Autodesk Inventor part; units mm, degrees
(part 6 of 13)
  spline S758 degree 3 poles (41.4277, 33.5866) (41.4277, 33.0506) (41.8622, 32.616) (42.3982, 32.616) knots 0 0 0 0 1 1 1 1
  line L2394 (41.4277, 33.5866) -> (41.4277, 33.0506) construction
  line L2395 (41.4277, 33.0506) -> (41.8622, 32.616) construction
  line L2396 (41.8622, 32.616) -> (42.3982, 32.616) construction
  spline S759 degree 3 poles (42.3982, 32.616) (42.9342, 32.616) (43.3688, 33.0506) (43.3688, 33.5866) knots 0 0 0 0 1 1 1 1
  line L2397 (42.3982, 32.616) -> (42.9342, 32.616) construction
  line L2398 (42.9342, 32.616) -> (43.3688, 33.0506) construction
  line L2399 (43.3688, 33.0506) -> (43.3688, 33.5866) construction
  spline S760 degree 3 poles (45.9229, 33.5866) (45.9229, 34.1226) (45.4883, 34.5571) (44.9523, 34.5571) knots 0 0 0 0 1 1 1 1
  line L2400 (45.9229, 33.5866) -> (45.9229, 34.1226) construction
  line L2401 (45.9229, 34.1226) -> (45.4883, 34.5571) construction
  line L2402 (45.4883, 34.5571) -> (44.9523, 34.5571) construction
  spline S761 degree 3 poles (44.9523, 34.5571) (44.4163, 34.5571) (43.9818, 34.1226) (43.9818, 33.5866) knots 0 0 0 0 1 1 1 1
  line L2403 (44.9523, 34.5571) -> (44.4163, 34.5571) construction
  line L2404 (44.4163, 34.5571) -> (43.9818, 34.1226) construction
  line L2405 (43.9818, 34.1226) -> (43.9818, 33.5866) construction
  spline S762 degree 3 poles (43.9818, 33.5866) (43.9818, 33.0506) (44.4163, 32.616) (44.9523, 32.616) knots 0 0 0 0 1 1 1 1
  line L2406 (43.9818, 33.5866) -> (43.9818, 33.0506) construction
  line L2407 (43.9818, 33.0506) -> (44.4163, 32.616) construction
  line L2408 (44.4163, 32.616) -> (44.9523, 32.616) construction
  spline S763 degree 3 poles (44.9523, 32.616) (45.4883, 32.616) (45.9229, 33.0506) (45.9229, 33.5866) knots 0 0 0 0 1 1 1 1
  line L2409 (44.9523, 32.616) -> (45.4883, 32.616) construction
  line L2410 (45.4883, 32.616) -> (45.9229, 33.0506) construction
  line L2411 (45.9229, 33.0506) -> (45.9229, 33.5866) construction
  spline S764 degree 3 poles (34.4294, 0.3832) (34.4294, 0.9191) (33.9948, 1.3537) (33.4588, 1.3537) knots 0 0 0 0 1 1 1 1
  line L2412 (34.4294, 0.3832) -> (34.4294, 0.9191) construction
  line L2413 (34.4294, 0.9191) -> (33.9948, 1.3537) construction
  line L2414 (33.9948, 1.3537) -> (33.4588, 1.3537) construction
  spline S765 degree 3 poles (33.4588, 1.3537) (32.9228, 1.3537) (32.4883, 0.9191) (32.4883, 0.3832) knots 0 0 0 0 1 1 1 1
  line L2415 (33.4588, 1.3537) -> (32.9228, 1.3537) construction
  line L2416 (32.9228, 1.3537) -> (32.4883, 0.9191) construction
  line L2417 (32.4883, 0.9191) -> (32.4883, 0.3832) construction
  spline S766 degree 3 poles (32.4883, 0.3832) (32.4883, -0.1529) (32.9228, -0.5874) (33.4588, -0.5874) knots 0 0 0 0 1 1 1 1
  line L2418 (32.4883, 0.3832) -> (32.4883, -0.1529) construction
  line L2419 (32.4883, -0.1529) -> (32.9228, -0.5874) construction
  line L2420 (32.9228, -0.5874) -> (33.4588, -0.5874) construction
  spline S767 degree 3 poles (33.4588, -0.5874) (33.9948, -0.5874) (34.4294, -0.1529) (34.4294, 0.3832) knots 0 0 0 0 1 1 1 1
  line L2421 (33.4588, -0.5874) -> (33.9948, -0.5874) construction
  line L2422 (33.9948, -0.5874) -> (34.4294, -0.1529) construction
  line L2423 (34.4294, -0.1529) -> (34.4294, 0.3832) construction
  spline S768 degree 3 poles (31.8752, 0.3832) (31.8752, 0.9191) (31.4407, 1.3537) (30.9047, 1.3537) knots 0 0 0 0 1 1 1 1
  line L2424 (31.8752, 0.3832) -> (31.8752, 0.9191) construction
  line L2425 (31.8752, 0.9191) -> (31.4407, 1.3537) construction
  line L2426 (31.4407, 1.3537) -> (30.9047, 1.3537) construction
  spline S769 degree 3 poles (30.9047, 1.3537) (30.3687, 1.3537) (29.9342, 0.9191) (29.9342, 0.3832) knots 0 0 0 0 1 1 1 1
  line L2427 (30.9047, 1.3537) -> (30.3687, 1.3537) construction
  line L2428 (30.3687, 1.3537) -> (29.9342, 0.9191) construction
  line L2429 (29.9342, 0.9191) -> (29.9342, 0.3832) construction
  spline S770 degree 3 poles (29.9342, 0.3832) (29.9342, -0.1529) (30.3687, -0.5874) (30.9047, -0.5874) knots 0 0 0 0 1 1 1 1
  line L2430 (29.9342, 0.3832) -> (29.9342, -0.1529) construction
  line L2431 (29.9342, -0.1529) -> (30.3687, -0.5874) construction
  line L2432 (30.3687, -0.5874) -> (30.9047, -0.5874) construction
  spline S771 degree 3 poles (30.9047, -0.5874) (31.4407, -0.5874) (31.8752, -0.1529) (31.8752, 0.3832) knots 0 0 0 0 1 1 1 1
  line L2433 (30.9047, -0.5874) -> (31.4407, -0.5874) construction
  line L2434 (31.4407, -0.5874) -> (31.8752, -0.1529) construction
  line L2435 (31.8752, -0.1529) -> (31.8752, 0.3832) construction
  spline S772 degree 3 poles (29.3211, 0.3832) (29.3211, 0.9191) (28.8866, 1.3537) (28.3506, 1.3537) knots 0 0 0 0 1 1 1 1
  line L2436 (29.3211, 0.3832) -> (29.3211, 0.9191) construction
  line L2437 (29.3211, 0.9191) -> (28.8866, 1.3537) construction
  line L2438 (28.8866, 1.3537) -> (28.3506, 1.3537) construction
  spline S773 degree 3 poles (28.3506, 1.3537) (27.8146, 1.3537) (27.3801, 0.9191) (27.3801, 0.3832) knots 0 0 0 0 1 1 1 1
  line L2439 (28.3506, 1.3537) -> (27.8146, 1.3537) construction
  line L2440 (27.8146, 1.3537) -> (27.3801, 0.9191) construction
  line L2441 (27.3801, 0.9191) -> (27.3801, 0.3832) construction
  spline S774 degree 3 poles (27.3801, 0.3832) (27.3801, -0.1529) (27.8146, -0.5874) (28.3506, -0.5874) knots 0 0 0 0 1 1 1 1
  line L2442 (27.3801, 0.3832) -> (27.3801, -0.1529) construction
  line L2443 (27.3801, -0.1529) -> (27.8146, -0.5874) construction
  line L2444 (27.8146, -0.5874) -> (28.3506, -0.5874) construction
  spline S775 degree 3 poles (28.3506, -0.5874) (28.8866, -0.5874) (29.3211, -0.1529) (29.3211, 0.3832) knots 0 0 0 0 1 1 1 1
  line L2445 (28.3506, -0.5874) -> (28.8866, -0.5874) construction
  line L2446 (28.8866, -0.5874) -> (29.3211, -0.1529) construction
  line L2447 (29.3211, -0.1529) -> (29.3211, 0.3832) construction
  spline S776 degree 3 poles (43.3688, 0.3832) (43.3688, 0.9191) (42.9342, 1.3537) (42.3982, 1.3537) knots 0 0 0 0 1 1 1 1
  line L2448 (43.3688, 0.3832) -> (43.3688, 0.9191) construction
  line L2449 (43.3688, 0.9191) -> (42.9342, 1.3537) construction
  line L2450 (42.9342, 1.3537) -> (42.3982, 1.3537) construction
  spline S777 degree 3 poles (42.3982, 1.3537) (41.8622, 1.3537) (41.4277, 0.9191) (41.4277, 0.3832) knots 0 0 0 0 1 1 1 1
  line L2451 (42.3982, 1.3537) -> (41.8622, 1.3537) construction
  line L2452 (41.8622, 1.3537) -> (41.4277, 0.9191) construction
  line L2453 (41.4277, 0.9191) -> (41.4277, 0.3832) construction
  spline S778 degree 3 poles (41.4277, 0.3832) (41.4277, -0.1529) (41.8622, -0.5874) (42.3982, -0.5874) knots 0 0 0 0 1 1 1 1
  line L2454 (41.4277, 0.3832) -> (41.4277, -0.1529) construction
  line L2455 (41.4277, -0.1529) -> (41.8622, -0.5874) construction
  line L2456 (41.8622, -0.5874) -> (42.3982, -0.5874) construction
  spline S779 degree 3 poles (42.3982, -0.5874) (42.9342, -0.5874) (43.3688, -0.1529) (43.3688, 0.3832) knots 0 0 0 0 1 1 1 1
  line L2457 (42.3982, -0.5874) -> (42.9342, -0.5874) construction
  line L2458 (42.9342, -0.5874) -> (43.3688, -0.1529) construction
  line L2459 (43.3688, -0.1529) -> (43.3688, 0.3832) construction
  spline S780 degree 3 poles (35.7064, 2.9373) (35.7064, 3.4732) (35.2719, 3.9078) (34.7358, 3.9078) knots 0 0 0 0 1 1 1 1
  line L2460 (35.7064, 2.9373) -> (35.7064, 3.4732) construction
  line L2461 (35.7064, 3.4732) -> (35.2719, 3.9078) construction
  line L2462 (35.2719, 3.9078) -> (34.7358, 3.9078) construction
  spline S781 degree 3 poles (34.7358, 3.9078) (34.1999, 3.9078) (33.7653, 3.4732) (33.7653, 2.9373) knots 0 0 0 0 1 1 1 1
  line L2463 (34.7358, 3.9078) -> (34.1999, 3.9078) construction
  line L2464 (34.1999, 3.9078) -> (33.7653, 3.4732) construction
  line L2465 (33.7653, 3.4732) -> (33.7653, 2.9373) construction
  spline S782 degree 3 poles (33.7653, 2.9373) (33.7653, 2.4013) (34.1999, 1.9667) (34.7358, 1.9667) knots 0 0 0 0 1 1 1 1
  line L2466 (33.7653, 2.9373) -> (33.7653, 2.4013) construction
  line L2467 (33.7653, 2.4013) -> (34.1999, 1.9667) construction
  line L2468 (34.1999, 1.9667) -> (34.7358, 1.9667) construction
  spline S783 degree 3 poles (34.7358, 1.9667) (35.2719, 1.9667) (35.7064, 2.4013) (35.7064, 2.9373) knots 0 0 0 0 1 1 1 1
  line L2469 (34.7358, 1.9667) -> (35.2719, 1.9667) construction
  line L2470 (35.2719, 1.9667) -> (35.7064, 2.4013) construction
  line L2471 (35.7064, 2.4013) -> (35.7064, 2.9373) construction
  spline S784 degree 3 poles (35.7064, 5.4914) (35.7064, 6.0273) (35.2719, 6.4619) (34.7358, 6.4619) knots 0 0 0 0 1 1 1 1
  line L2472 (35.7064, 5.4914) -> (35.7064, 6.0273) construction
  line L2473 (35.7064, 6.0273) -> (35.2719, 6.4619) construction
  line L2474 (35.2719, 6.4619) -> (34.7358, 6.4619) construction
  spline S785 degree 3 poles (34.7358, 6.4619) (34.1999, 6.4619) (33.7653, 6.0273) (33.7653, 5.4914) knots 0 0 0 0 1 1 1 1
  line L2475 (34.7358, 6.4619) -> (34.1999, 6.4619) construction
  line L2476 (34.1999, 6.4619) -> (33.7653, 6.0273) construction
  line L2477 (33.7653, 6.0273) -> (33.7653, 5.4914) construction
  spline S786 degree 3 poles (33.7653, 5.4914) (33.7653, 4.9554) (34.1999, 4.5208) (34.7358, 4.5208) knots 0 0 0 0 1 1 1 1
  line L2478 (33.7653, 5.4914) -> (33.7653, 4.9554) construction
  line L2479 (33.7653, 4.9554) -> (34.1999, 4.5208) construction
  line L2480 (34.1999, 4.5208) -> (34.7358, 4.5208) construction
  spline S787 degree 3 poles (34.7358, 4.5208) (35.2719, 4.5208) (35.7064, 4.9554) (35.7064, 5.4914) knots 0 0 0 0 1 1 1 1
  line L2481 (34.7358, 4.5208) -> (35.2719, 4.5208) construction
  line L2482 (35.2719, 4.5208) -> (35.7064, 4.9554) construction
  line L2483 (35.7064, 4.9554) -> (35.7064, 5.4914) construction
  spline S788 degree 3 poles (38.2606, 5.4914) (38.2606, 6.0273) (37.826, 6.4619) (37.29, 6.4619) knots 0 0 0 0 1 1 1 1
  line L2484 (38.2606, 5.4914) -> (38.2606, 6.0273) construction
  line L2485 (38.2606, 6.0273) -> (37.826, 6.4619) construction
  line L2486 (37.826, 6.4619) -> (37.29, 6.4619) construction
  spline S789 degree 3 poles (37.29, 6.4619) (36.754, 6.4619) (36.3194, 6.0273) (36.3194, 5.4914) knots 0 0 0 0 1 1 1 1
  line L2487 (37.29, 6.4619) -> (36.754, 6.4619) construction
  line L2488 (36.754, 6.4619) -> (36.3194, 6.0273) construction
  line L2489 (36.3194, 6.0273) -> (36.3194, 5.4914) construction
  spline S790 degree 3 poles (36.3194, 5.4914) (36.3194, 4.9554) (36.754, 4.5208) (37.29, 4.5208) knots 0 0 0 0 1 1 1 1
  line L2490 (36.3194, 5.4914) -> (36.3194, 4.9554) construction
  line L2491 (36.3194, 4.9554) -> (36.754, 4.5208) construction
  line L2492 (36.754, 4.5208) -> (37.29, 4.5208) construction
  spline S791 degree 3 poles (37.29, 4.5208) (37.826, 4.5208) (38.2606, 4.9554) (38.2606, 5.4914) knots 0 0 0 0 1 1 1 1
  line L2493 (37.29, 4.5208) -> (37.826, 4.5208) construction
  line L2494 (37.826, 4.5208) -> (38.2606, 4.9554) construction
  line L2495 (38.2606, 4.9554) -> (38.2606, 5.4914) construction
  spline S792 degree 3 poles (38.2606, 0.3832) (38.2606, 0.9191) (37.826, 1.3537) (37.29, 1.3537) knots 0 0 0 0 1 1 1 1
  line L2496 (38.2606, 0.3832) -> (38.2606, 0.9191) construction
  line L2497 (38.2606, 0.9191) -> (37.826, 1.3537) construction
  line L2498 (37.826, 1.3537) -> (37.29, 1.3537) construction
  spline S793 degree 3 poles (37.29, 1.3537) (36.754, 1.3537) (36.3194, 0.9191) (36.3194, 0.3832) knots 0 0 0 0 1 1 1 1
  line L2499 (37.29, 1.3537) -> (36.754, 1.3537) construction
  line L2500 (36.754, 1.3537) -> (36.3194, 0.9191) construction
  line L2501 (36.3194, 0.9191) -> (36.3194, 0.3832) construction
  spline S794 degree 3 poles (36.3194, 0.3832) (36.3194, -0.1529) (36.754, -0.5874) (37.29, -0.5874) knots 0 0 0 0 1 1 1 1
  line L2502 (36.3194, 0.3832) -> (36.3194, -0.1529) construction
  line L2503 (36.3194, -0.1529) -> (36.754, -0.5874) construction
  line L2504 (36.754, -0.5874) -> (37.29, -0.5874) construction
  spline S795 degree 3 poles (37.29, -0.5874) (37.826, -0.5874) (38.2606, -0.1529) (38.2606, 0.3832) knots 0 0 0 0 1 1 1 1
  line L2505 (37.29, -0.5874) -> (37.826, -0.5874) construction
  line L2506 (37.826, -0.5874) -> (38.2606, -0.1529) construction
  line L2507 (38.2606, -0.1529) -> (38.2606, 0.3832) construction
  spline S796 degree 3 poles (40.8147, 0.3832) (40.8147, 0.9191) (40.3801, 1.3537) (39.8441, 1.3537) knots 0 0 0 0 1 1 1 1
  line L2508 (40.8147, 0.3832) -> (40.8147, 0.9191) construction
  line L2509 (40.8147, 0.9191) -> (40.3801, 1.3537) construction
  line L2510 (40.3801, 1.3537) -> (39.8441, 1.3537) construction
  spline S797 degree 3 poles (39.8441, 1.3537) (39.3081, 1.3537) (38.8735, 0.9191) (38.8735, 0.3832) knots 0 0 0 0 1 1 1 1
  line L2511 (39.8441, 1.3537) -> (39.3081, 1.3537) construction
  line L2512 (39.3081, 1.3537) -> (38.8735, 0.9191) construction
  line L2513 (38.8735, 0.9191) -> (38.8735, 0.3832) construction
  spline S798 degree 3 poles (38.8735, 0.3832) (38.8735, -0.1529) (39.3081, -0.5874) (39.8441, -0.5874) knots 0 0 0 0 1 1 1 1
  line L2514 (38.8735, 0.3832) -> (38.8735, -0.1529) construction
  line L2515 (38.8735, -0.1529) -> (39.3081, -0.5874) construction
  line L2516 (39.3081, -0.5874) -> (39.8441, -0.5874) construction
  spline S799 degree 3 poles (39.8441, -0.5874) (40.3801, -0.5874) (40.8147, -0.1529) (40.8147, 0.3832) knots 0 0 0 0 1 1 1 1
  line L2517 (39.8441, -0.5874) -> (40.3801, -0.5874) construction
  line L2518 (40.3801, -0.5874) -> (40.8147, -0.1529) construction
  line L2519 (40.8147, -0.1529) -> (40.8147, 0.3832) construction
  spline S800 degree 3 poles (38.2606, 2.9373) (38.2606, 3.4732) (37.826, 3.9078) (37.29, 3.9078) knots 0 0 0 0 1 1 1 1
  line L2520 (38.2606, 2.9373) -> (38.2606, 3.4732) construction
  line L2521 (38.2606, 3.4732) -> (37.826, 3.9078) construction
  line L2522 (37.826, 3.9078) -> (37.29, 3.9078) construction
  spline S801 degree 3 poles (37.29, 3.9078) (36.754, 3.9078) (36.3194, 3.4732) (36.3194, 2.9373) knots 0 0 0 0 1 1 1 1
  line L2523 (37.29, 3.9078) -> (36.754, 3.9078) construction
  line L2524 (36.754, 3.9078) -> (36.3194, 3.4732) construction
  line L2525 (36.3194, 3.4732) -> (36.3194, 2.9373) construction
  spline S802 degree 3 poles (36.3194, 2.9373) (36.3194, 2.4013) (36.754, 1.9667) (37.29, 1.9667) knots 0 0 0 0 1 1 1 1
  line L2526 (36.3194, 2.9373) -> (36.3194, 2.4013) construction
  line L2527 (36.3194, 2.4013) -> (36.754, 1.9667) construction
  line L2528 (36.754, 1.9667) -> (37.29, 1.9667) construction
  spline S803 degree 3 poles (37.29, 1.9667) (37.826, 1.9667) (38.2606, 2.4013) (38.2606, 2.9373) knots 0 0 0 0 1 1 1 1
  line L2529 (37.29, 1.9667) -> (37.826, 1.9667) construction
  line L2530 (37.826, 1.9667) -> (38.2606, 2.4013) construction
  line L2531 (38.2606, 2.4013) -> (38.2606, 2.9373) construction
  spline S804 degree 3 poles (35.7064, 8.0455) (35.7064, 8.5815) (35.2719, 9.016) (34.7358, 9.016) knots 0 0 0 0 1 1 1 1
  line L2532 (35.7064, 8.0455) -> (35.7064, 8.5815) construction
  line L2533 (35.7064, 8.5815) -> (35.2719, 9.016) construction
  line L2534 (35.2719, 9.016) -> (34.7358, 9.016) construction
  spline S805 degree 3 poles (34.7358, 9.016) (34.1999, 9.016) (33.7653, 8.5815) (33.7653, 8.0455) knots 0 0 0 0 1 1 1 1
  line L2535 (34.7358, 9.016) -> (34.1999, 9.016) construction
  line L2536 (34.1999, 9.016) -> (33.7653, 8.5815) construction
  line L2537 (33.7653, 8.5815) -> (33.7653, 8.0455) construction
  spline S806 degree 3 poles (33.7653, 8.0455) (33.7653, 7.5095) (34.1999, 7.0749) (34.7358, 7.0749) knots 0 0 0 0 1 1 1 1
  line L2538 (33.7653, 8.0455) -> (33.7653, 7.5095) construction
  line L2539 (33.7653, 7.5095) -> (34.1999, 7.0749) construction
  line L2540 (34.1999, 7.0749) -> (34.7358, 7.0749) construction
  spline S807 degree 3 poles (34.7358, 7.0749) (35.2719, 7.0749) (35.7064, 7.5095) (35.7064, 8.0455) knots 0 0 0 0 1 1 1 1
  line L2541 (34.7358, 7.0749) -> (35.2719, 7.0749) construction
  line L2542 (35.2719, 7.0749) -> (35.7064, 7.5095) construction
  line L2543 (35.7064, 7.5095) -> (35.7064, 8.0455) construction
  spline S808 degree 3 poles (38.2606, 8.0455) (38.2606, 8.5815) (37.826, 9.016) (37.29, 9.016) knots 0 0 0 0 1 1 1 1
  line L2544 (38.2606, 8.0455) -> (38.2606, 8.5815) construction
  line L2545 (38.2606, 8.5815) -> (37.826, 9.016) construction
  line L2546 (37.826, 9.016) -> (37.29, 9.016) construction
  spline S809 degree 3 poles (37.29, 9.016) (36.754, 9.016) (36.3194, 8.5815) (36.3194, 8.0455) knots 0 0 0 0 1 1 1 1
  line L2547 (37.29, 9.016) -> (36.754, 9.016) construction
  line L2548 (36.754, 9.016) -> (36.3194, 8.5815) construction
  line L2549 (36.3194, 8.5815) -> (36.3194, 8.0455) construction
  spline S810 degree 3 poles (36.3194, 8.0455) (36.3194, 7.5095) (36.754, 7.0749) (37.29, 7.0749) knots 0 0 0 0 1 1 1 1
  line L2550 (36.3194, 8.0455) -> (36.3194, 7.5095) construction
  line L2551 (36.3194, 7.5095) -> (36.754, 7.0749) construction
  line L2552 (36.754, 7.0749) -> (37.29, 7.0749) construction
  spline S811 degree 3 poles (37.29, 7.0749) (37.826, 7.0749) (38.2606, 7.5095) (38.2606, 8.0455) knots 0 0 0 0 1 1 1 1
  line L2553 (37.29, 7.0749) -> (37.826, 7.0749) construction
  line L2554 (37.826, 7.0749) -> (38.2606, 7.5095) construction
  line L2555 (38.2606, 7.5095) -> (38.2606, 8.0455) construction
  spline S812 degree 3 poles (35.7064, 10.5996) (35.7064, 11.1356) (35.2719, 11.5701) (34.7358, 11.5701) knots 0 0 0 0 1 1 1 1
  line L2556 (35.7064, 10.5996) -> (35.7064, 11.1356) construction
  line L2557 (35.7064, 11.1356) -> (35.2719, 11.5701) construction
  line L2558 (35.2719, 11.5701) -> (34.7358, 11.5701) construction
  spline S813 degree 3 poles (34.7358, 11.5701) (34.1999, 11.5701) (33.7653, 11.1356) (33.7653, 10.5996) knots 0 0 0 0 1 1 1 1
  line L2559 (34.7358, 11.5701) -> (34.1999, 11.5701) construction
  line L2560 (34.1999, 11.5701) -> (33.7653, 11.1356) construction
  line L2561 (33.7653, 11.1356) -> (33.7653, 10.5996) construction
  spline S814 degree 3 poles (33.7653, 10.5996) (33.7653, 10.0636) (34.1999, 9.629) (34.7358, 9.629) knots 0 0 0 0 1 1 1 1
  line L2562 (33.7653, 10.5996) -> (33.7653, 10.0636) construction
  line L2563 (33.7653, 10.0636) -> (34.1999, 9.629) construction
  line L2564 (34.1999, 9.629) -> (34.7358, 9.629) construction
  spline S815 degree 3 poles (34.7358, 9.629) (35.2719, 9.629) (35.7064, 10.0636) (35.7064, 10.5996) knots 0 0 0 0 1 1 1 1
  line L2565 (34.7358, 9.629) -> (35.2719, 9.629) construction
  line L2566 (35.2719, 9.629) -> (35.7064, 10.0636) construction
  line L2567 (35.7064, 10.0636) -> (35.7064, 10.5996) construction
  spline S816 degree 3 poles (38.2606, 10.5996) (38.2606, 11.1356) (37.826, 11.5701) (37.29, 11.5701) knots 0 0 0 0 1 1 1 1
  line L2568 (38.2606, 10.5996) -> (38.2606, 11.1356) construction
  line L2569 (38.2606, 11.1356) -> (37.826, 11.5701) construction
  line L2570 (37.826, 11.5701) -> (37.29, 11.5701) construction
  spline S817 degree 3 poles (37.29, 11.5701) (36.754, 11.5701) (36.3194, 11.1356) (36.3194, 10.5996) knots 0 0 0 0 1 1 1 1
  line L2571 (37.29, 11.5701) -> (36.754, 11.5701) construction
  line L2572 (36.754, 11.5701) -> (36.3194, 11.1356) construction
  line L2573 (36.3194, 11.1356) -> (36.3194, 10.5996) construction
  spline S818 degree 3 poles (36.3194, 10.5996) (36.3194, 10.0636) (36.754, 9.629) (37.29, 9.629) knots 0 0 0 0 1 1 1 1
  line L2574 (36.3194, 10.5996) -> (36.3194, 10.0636) construction
  line L2575 (36.3194, 10.0636) -> (36.754, 9.629) construction
  line L2576 (36.754, 9.629) -> (37.29, 9.629) construction
  spline S819 degree 3 poles (37.29, 9.629) (37.826, 9.629) (38.2606, 10.0636) (38.2606, 10.5996) knots 0 0 0 0 1 1 1 1
  line L2577 (37.29, 9.629) -> (37.826, 9.629) construction
  line L2578 (37.826, 9.629) -> (38.2606, 10.0636) construction
  line L2579 (38.2606, 10.0636) -> (38.2606, 10.5996) construction
  spline S820 degree 3 poles (35.7064, 13.1537) (35.7064, 13.6897) (35.2719, 14.1242) (34.7358, 14.1242) knots 0 0 0 0 1 1 1 1
  line L2580 (35.7064, 13.1537) -> (35.7064, 13.6897) construction
  line L2581 (35.7064, 13.6897) -> (35.2719, 14.1242) construction
  line L2582 (35.2719, 14.1242) -> (34.7358, 14.1242) construction
  spline S821 degree 3 poles (34.7358, 14.1242) (34.1999, 14.1242) (33.7653, 13.6897) (33.7653, 13.1537) knots 0 0 0 0 1 1 1 1
  line L2583 (34.7358, 14.1242) -> (34.1999, 14.1242) construction
  line L2584 (34.1999, 14.1242) -> (33.7653, 13.6897) construction
  line L2585 (33.7653, 13.6897) -> (33.7653, 13.1537) construction
  spline S822 degree 3 poles (33.7653, 13.1537) (33.7653, 12.6177) (34.1999, 12.1831) (34.7358, 12.1831) knots 0 0 0 0 1 1 1 1
  line L2586 (33.7653, 13.1537) -> (33.7653, 12.6177) construction
  line L2587 (33.7653, 12.6177) -> (34.1999, 12.1831) construction
  line L2588 (34.1999, 12.1831) -> (34.7358, 12.1831) construction
  spline S823 degree 3 poles (34.7358, 12.1831) (35.2719, 12.1831) (35.7064, 12.6177) (35.7064, 13.1537) knots 0 0 0 0 1 1 1 1
  line L2589 (34.7358, 12.1831) -> (35.2719, 12.1831) construction
  line L2590 (35.2719, 12.1831) -> (35.7064, 12.6177) construction
  line L2591 (35.7064, 12.6177) -> (35.7064, 13.1537) construction
  spline S824 degree 3 poles (38.2606, 13.1537) (38.2606, 13.6897) (37.826, 14.1242) (37.29, 14.1242) knots 0 0 0 0 1 1 1 1
  line L2592 (38.2606, 13.1537) -> (38.2606, 13.6897) construction
  line L2593 (38.2606, 13.6897) -> (37.826, 14.1242) construction
  line L2594 (37.826, 14.1242) -> (37.29, 14.1242) construction
  spline S825 degree 3 poles (37.29, 14.1242) (36.754, 14.1242) (36.3194, 13.6897) (36.3194, 13.1537) knots 0 0 0 0 1 1 1 1
  line L2595 (37.29, 14.1242) -> (36.754, 14.1242) construction
  line L2596 (36.754, 14.1242) -> (36.3194, 13.6897) construction
  line L2597 (36.3194, 13.6897) -> (36.3194, 13.1537) construction
  spline S826 degree 3 poles (36.3194, 13.1537) (36.3194, 12.6177) (36.754, 12.1831) (37.29, 12.1831) knots 0 0 0 0 1 1 1 1
  line L2598 (36.3194, 13.1537) -> (36.3194, 12.6177) construction
  line L2599 (36.3194, 12.6177) -> (36.754, 12.1831) construction
  line L2600 (36.754, 12.1831) -> (37.29, 12.1831) construction
  spline S827 degree 3 poles (37.29, 12.1831) (37.826, 12.1831) (38.2606, 12.6177) (38.2606, 13.1537) knots 0 0 0 0 1 1 1 1
  line L2601 (37.29, 12.1831) -> (37.826, 12.1831) construction
  line L2602 (37.826, 12.1831) -> (38.2606, 12.6177) construction
  line L2603 (38.2606, 12.6177) -> (38.2606, 13.1537) construction
  spline S828 degree 3 poles (35.7064, 15.7078) (35.7064, 16.2438) (35.2719, 16.6783) (34.7358, 16.6783) knots 0 0 0 0 1 1 1 1
  line L2604 (35.7064, 15.7078) -> (35.7064, 16.2438) construction
  line L2605 (35.7064, 16.2438) -> (35.2719, 16.6783) construction
  line L2606 (35.2719, 16.6783) -> (34.7358, 16.6783) construction
  spline S829 degree 3 poles (34.7358, 16.6783) (34.1999, 16.6783) (33.7653, 16.2438) (33.7653, 15.7078) knots 0 0 0 0 1 1 1 1
  line L2607 (34.7358, 16.6783) -> (34.1999, 16.6783) construction
  line L2608 (34.1999, 16.6783) -> (33.7653, 16.2438) construction
  line L2609 (33.7653, 16.2438) -> (33.7653, 15.7078) construction
  spline S830 degree 3 poles (33.7653, 15.7078) (33.7653, 15.1718) (34.1999, 14.7372) (34.7358, 14.7372) knots 0 0 0 0 1 1 1 1
  line L2610 (33.7653, 15.7078) -> (33.7653, 15.1718) construction
  line L2611 (33.7653, 15.1718) -> (34.1999, 14.7372) construction
  line L2612 (34.1999, 14.7372) -> (34.7358, 14.7372) construction
  spline S831 degree 3 poles (34.7358, 14.7372) (35.2719, 14.7372) (35.7064, 15.1718) (35.7064, 15.7078) knots 0 0 0 0 1 1 1 1
  line L2613 (34.7358, 14.7372) -> (35.2719, 14.7372) construction
  line L2614 (35.2719, 14.7372) -> (35.7064, 15.1718) construction
  line L2615 (35.7064, 15.1718) -> (35.7064, 15.7078) construction
  spline S832 degree 3 poles (38.2606, 15.7078) (38.2606, 16.2438) (37.826, 16.6783) (37.29, 16.6783) knots 0 0 0 0 1 1 1 1
  line L2616 (38.2606, 15.7078) -> (38.2606, 16.2438) construction
  line L2617 (38.2606, 16.2438) -> (37.826, 16.6783) construction
  line L2618 (37.826, 16.6783) -> (37.29, 16.6783) construction
  spline S833 degree 3 poles (37.29, 16.6783) (36.754, 16.6783) (36.3194, 16.2438) (36.3194, 15.7078) knots 0 0 0 0 1 1 1 1
  line L2619 (37.29, 16.6783) -> (36.754, 16.6783) construction
  line L2620 (36.754, 16.6783) -> (36.3194, 16.2438) construction
  line L2621 (36.3194, 16.2438) -> (36.3194, 15.7078) construction
  spline S834 degree 3 poles (36.3194, 15.7078) (36.3194, 15.1718) (36.754, 14.7372) (37.29, 14.7372) knots 0 0 0 0 1 1 1 1
  line L2622 (36.3194, 15.7078) -> (36.3194, 15.1718) construction
  line L2623 (36.3194, 15.1718) -> (36.754, 14.7372) construction
  line L2624 (36.754, 14.7372) -> (37.29, 14.7372) construction
  spline S835 degree 3 poles (37.29, 14.7372) (37.826, 14.7372) (38.2606, 15.1718) (38.2606, 15.7078) knots 0 0 0 0 1 1 1 1
  line L2625 (37.29, 14.7372) -> (37.826, 14.7372) construction
  line L2626 (37.826, 14.7372) -> (38.2606, 15.1718) construction
  line L2627 (38.2606, 15.1718) -> (38.2606, 15.7078) construction
  spline S836 degree 3 poles (35.7064, 18.2619) (35.7064, 18.7979) (35.2719, 19.2324) (34.7358, 19.2324) knots 0 0 0 0 1 1 1 1
  line L2628 (35.7064, 18.2619) -> (35.7064, 18.7979) construction
  line L2629 (35.7064, 18.7979) -> (35.2719, 19.2324) construction
  line L2630 (35.2719, 19.2324) -> (34.7358, 19.2324) construction
  spline S837 degree 3 poles (34.7358, 19.2324) (34.1999, 19.2324) (33.7653, 18.7979) (33.7653, 18.2619) knots 0 0 0 0 1 1 1 1
  line L2631 (34.7358, 19.2324) -> (34.1999, 19.2324) construction
  line L2632 (34.1999, 19.2324) -> (33.7653, 18.7979) construction
  line L2633 (33.7653, 18.7979) -> (33.7653, 18.2619) construction
  spline S838 degree 3 poles (33.7653, 18.2619) (33.7653, 17.7259) (34.1999, 17.2914) (34.7358, 17.2914) knots 0 0 0 0 1 1 1 1
  line L2634 (33.7653, 18.2619) -> (33.7653, 17.7259) construction
  line L2635 (33.7653, 17.7259) -> (34.1999, 17.2914) construction
  line L2636 (34.1999, 17.2914) -> (34.7358, 17.2914) construction
  spline S839 degree 3 poles (34.7358, 17.2914) (35.2719, 17.2914) (35.7064, 17.7259) (35.7064, 18.2619) knots 0 0 0 0 1 1 1 1
  line L2637 (34.7358, 17.2914) -> (35.2719, 17.2914) construction
  line L2638 (35.2719, 17.2914) -> (35.7064, 17.7259) construction
  line L2639 (35.7064, 17.7259) -> (35.7064, 18.2619) construction
  spline S840 degree 3 poles (38.2606, 18.2619) (38.2606, 18.7979) (37.826, 19.2324) (37.29, 19.2324) knots 0 0 0 0 1 1 1 1
  line L2640 (38.2606, 18.2619) -> (38.2606, 18.7979) construction
  line L2641 (38.2606, 18.7979) -> (37.826, 19.2324) construction
  line L2642 (37.826, 19.2324) -> (37.29, 19.2324) construction
  spline S841 degree 3 poles (37.29, 19.2324) (36.754, 19.2324) (36.3194, 18.7979) (36.3194, 18.2619) knots 0 0 0 0 1 1 1 1
  line L2643 (37.29, 19.2324) -> (36.754, 19.2324) construction
  line L2644 (36.754, 19.2324) -> (36.3194, 18.7979) construction
  line L2645 (36.3194, 18.7979) -> (36.3194, 18.2619) construction
  spline S842 degree 3 poles (36.3194, 18.2619) (36.3194, 17.7259) (36.754, 17.2914) (37.29, 17.2914) knots 0 0 0 0 1 1 1 1
  line L2646 (36.3194, 18.2619) -> (36.3194, 17.7259) construction
  line L2647 (36.3194, 17.7259) -> (36.754, 17.2914) construction
  line L2648 (36.754, 17.2914) -> (37.29, 17.2914) construction
  spline S843 degree 3 poles (37.29, 17.2914) (37.826, 17.2914) (38.2606, 17.7259) (38.2606, 18.2619) knots 0 0 0 0 1 1 1 1
  line L2649 (37.29, 17.2914) -> (37.826, 17.2914) construction
  line L2650 (37.826, 17.2914) -> (38.2606, 17.7259) construction
  line L2651 (38.2606, 17.7259) -> (38.2606, 18.2619) construction
  spline S844 degree 3 poles (35.7064, 20.816) (35.7064, 21.352) (35.2719, 21.7866) (34.7358, 21.7866) knots 0 0 0 0 1 1 1 1
  line L2652 (35.7064, 20.816) -> (35.7064, 21.352) construction
  line L2653 (35.7064, 21.352) -> (35.2719, 21.7866) construction
  line L2654 (35.2719, 21.7866) -> (34.7358, 21.7866) construction
  spline S845 degree 3 poles (34.7358, 21.7866) (34.1999, 21.7866) (33.7653, 21.352) (33.7653, 20.816) knots 0 0 0 0 1 1 1 1
  line L2655 (34.7358, 21.7866) -> (34.1999, 21.7866) construction
  line L2656 (34.1999, 21.7866) -> (33.7653, 21.352) construction
  line L2657 (33.7653, 21.352) -> (33.7653, 20.816) construction
  spline S846 degree 3 poles (33.7653, 20.816) (33.7653, 20.28) (34.1999, 19.8455) (34.7358, 19.8455) knots 0 0 0 0 1 1 1 1
  line L2658 (33.7653, 20.816) -> (33.7653, 20.28) construction
  line L2659 (33.7653, 20.28) -> (34.1999, 19.8455) construction
  line L2660 (34.1999, 19.8455) -> (34.7358, 19.8455) construction
  spline S847 degree 3 poles (34.7358, 19.8455) (35.2719, 19.8455) (35.7064, 20.28) (35.7064, 20.816) knots 0 0 0 0 1 1 1 1
  line L2661 (34.7358, 19.8455) -> (35.2719, 19.8455) construction
  line L2662 (35.2719, 19.8455) -> (35.7064, 20.28) construction
  line L2663 (35.7064, 20.28) -> (35.7064, 20.816) construction
  spline S848 degree 3 poles (35.7064, 23.3701) (35.7064, 23.9061) (35.2719, 24.3407) (34.7358, 24.3407) knots 0 0 0 0 1 1 1 1
  line L2664 (35.7064, 23.3701) -> (35.7064, 23.9061) construction
  line L2665 (35.7064, 23.9061) -> (35.2719, 24.3407) construction
  line L2666 (35.2719, 24.3407) -> (34.7358, 24.3407) construction
  spline S849 degree 3 poles (34.7358, 24.3407) (34.1999, 24.3407) (33.7653, 23.9061) (33.7653, 23.3701) knots 0 0 0 0 1 1 1 1
  line L2667 (34.7358, 24.3407) -> (34.1999, 24.3407) construction
  line L2668 (34.1999, 24.3407) -> (33.7653, 23.9061) construction
  line L2669 (33.7653, 23.9061) -> (33.7653, 23.3701) construction
  spline S850 degree 3 poles (33.7653, 23.3701) (33.7653, 22.8341) (34.1999, 22.3996) (34.7358, 22.3996) knots 0 0 0 0 1 1 1 1
  line L2670 (33.7653, 23.3701) -> (33.7653, 22.8341) construction
  line L2671 (33.7653, 22.8341) -> (34.1999, 22.3996) construction
  line L2672 (34.1999, 22.3996) -> (34.7358, 22.3996) construction
  spline S851 degree 3 poles (34.7358, 22.3996) (35.2719, 22.3996) (35.7064, 22.8341) (35.7064, 23.3701) knots 0 0 0 0 1 1 1 1
  line L2673 (34.7358, 22.3996) -> (35.2719, 22.3996) construction
  line L2674 (35.2719, 22.3996) -> (35.7064, 22.8341) construction
  line L2675 (35.7064, 22.8341) -> (35.7064, 23.3701) construction
  spline S852 degree 3 poles (35.7064, 25.9242) (35.7064, 26.4602) (35.2719, 26.8948) (34.7358, 26.8948) knots 0 0 0 0 1 1 1 1
  line L2676 (35.7064, 25.9242) -> (35.7064, 26.4602) construction
  line L2677 (35.7064, 26.4602) -> (35.2719, 26.8948) construction
  line L2678 (35.2719, 26.8948) -> (34.7358, 26.8948) construction
  spline S853 degree 3 poles (34.7358, 26.8948) (34.1999, 26.8948) (33.7653, 26.4602) (33.7653, 25.9242) knots 0 0 0 0 1 1 1 1
  line L2679 (34.7358, 26.8948) -> (34.1999, 26.8948) construction
  line L2680 (34.1999, 26.8948) -> (33.7653, 26.4602) construction
  line L2681 (33.7653, 26.4602) -> (33.7653, 25.9242) construction
  spline S854 degree 3 poles (33.7653, 25.9242) (33.7653, 25.3882) (34.1999, 24.9537) (34.7358, 24.9537) knots 0 0 0 0 1 1 1 1
  line L2682 (33.7653, 25.9242) -> (33.7653, 25.3882) construction
  line L2683 (33.7653, 25.3882) -> (34.1999, 24.9537) construction
  line L2684 (34.1999, 24.9537) -> (34.7358, 24.9537) construction
  spline S855 degree 3 poles (34.7358, 24.9537) (35.2719, 24.9537) (35.7064, 25.3882) (35.7064, 25.9242) knots 0 0 0 0 1 1 1 1
  line L2685 (34.7358, 24.9537) -> (35.2719, 24.9537) construction
  line L2686 (35.2719, 24.9537) -> (35.7064, 25.3882) construction
  line L2687 (35.7064, 25.3882) -> (35.7064, 25.9242) construction
  spline S856 degree 3 poles (35.7064, 28.4784) (35.7064, 29.0143) (35.2719, 29.4489) (34.7358, 29.4489) knots 0 0 0 0 1 1 1 1
  line L2688 (35.7064, 28.4784) -> (35.7064, 29.0143) construction
  line L2689 (35.7064, 29.0143) -> (35.2719, 29.4489) construction
  line L2690 (35.2719, 29.4489) -> (34.7358, 29.4489) construction
  spline S857 degree 3 poles (34.7358, 29.4489) (34.1999, 29.4489) (33.7653, 29.0143) (33.7653, 28.4784) knots 0 0 0 0 1 1 1 1
  line L2691 (34.7358, 29.4489) -> (34.1999, 29.4489) construction
  line L2692 (34.1999, 29.4489) -> (33.7653, 29.0143) construction
  line L2693 (33.7653, 29.0143) -> (33.7653, 28.4784) construction
  spline S858 degree 3 poles (33.7653, 28.4784) (33.7653, 27.9423) (34.1999, 27.5078) (34.7358, 27.5078) knots 0 0 0 0 1 1 1 1
  line L2694 (33.7653, 28.4784) -> (33.7653, 27.9423) construction
  line L2695 (33.7653, 27.9423) -> (34.1999, 27.5078) construction
  line L2696 (34.1999, 27.5078) -> (34.7358, 27.5078) construction
  spline S859 degree 3 poles (34.7358, 27.5078) (35.2719, 27.5078) (35.7064, 27.9423) (35.7064, 28.4784) knots 0 0 0 0 1 1 1 1
  line L2697 (34.7358, 27.5078) -> (35.2719, 27.5078) construction
  line L2698 (35.2719, 27.5078) -> (35.7064, 27.9423) construction
  line L2699 (35.7064, 27.9423) -> (35.7064, 28.4784) construction
  spline S860 degree 3 poles (35.7064, 31.0325) (35.7064, 31.5684) (35.2719, 32.003) (34.7358, 32.003) knots 0 0 0 0 1 1 1 1
  line L2700 (35.7064, 31.0325) -> (35.7064, 31.5684) construction
  line L2701 (35.7064, 31.5684) -> (35.2719, 32.003) construction
  line L2702 (35.2719, 32.003) -> (34.7358, 32.003) construction
  spline S861 degree 3 poles (34.7358, 32.003) (34.1999, 32.003) (33.7653, 31.5684) (33.7653, 31.0325) knots 0 0 0 0 1 1 1 1
  line L2703 (34.7358, 32.003) -> (34.1999, 32.003) construction
  line L2704 (34.1999, 32.003) -> (33.7653, 31.5684) construction
  line L2705 (33.7653, 31.5684) -> (33.7653, 31.0325) construction
  spline S862 degree 3 poles (33.7653, 31.0325) (33.7653, 30.4965) (34.1999, 30.0619) (34.7358, 30.0619) knots 0 0 0 0 1 1 1 1
  line L2706 (33.7653, 31.0325) -> (33.7653, 30.4965) construction
  line L2707 (33.7653, 30.4965) -> (34.1999, 30.0619) construction
  line L2708 (34.1999, 30.0619) -> (34.7358, 30.0619) construction
  spline S863 degree 3 poles (34.7358, 30.0619) (35.2719, 30.0619) (35.7064, 30.4965) (35.7064, 31.0325) knots 0 0 0 0 1 1 1 1
  line L2709 (34.7358, 30.0619) -> (35.2719, 30.0619) construction
  line L2710 (35.2719, 30.0619) -> (35.7064, 30.4965) construction
  line L2711 (35.7064, 30.4965) -> (35.7064, 31.0325) construction
  spline S864 degree 3 poles (38.2606, 20.816) (38.2606, 21.352) (37.826, 21.7866) (37.29, 21.7866) knots 0 0 0 0 1 1 1 1
  line L2712 (38.2606, 20.816) -> (38.2606, 21.352) construction
  line L2713 (38.2606, 21.352) -> (37.826, 21.7866) construction
  line L2714 (37.826, 21.7866) -> (37.29, 21.7866) construction
  spline S865 degree 3 poles (37.29, 21.7866) (36.754, 21.7866) (36.3194, 21.352) (36.3194, 20.816) knots 0 0 0 0 1 1 1 1
  line L2715 (37.29, 21.7866) -> (36.754, 21.7866) construction
  line L2716 (36.754, 21.7866) -> (36.3194, 21.352) construction
  line L2717 (36.3194, 21.352) -> (36.3194, 20.816) construction
  spline S866 degree 3 poles (36.3194, 20.816) (36.3194, 20.28) (36.754, 19.8455) (37.29, 19.8455) knots 0 0 0 0 1 1 1 1
  line L2718 (36.3194, 20.816) -> (36.3194, 20.28) construction
  line L2719 (36.3194, 20.28) -> (36.754, 19.8455) construction
  line L2720 (36.754, 19.8455) -> (37.29, 19.8455) construction
  spline S867 degree 3 poles (37.29, 19.8455) (37.826, 19.8455) (38.2606, 20.28) (38.2606, 20.816) knots 0 0 0 0 1 1 1 1
  line L2721 (37.29, 19.8455) -> (37.826, 19.8455) construction
  line L2722 (37.826, 19.8455) -> (38.2606, 20.28) construction
  line L2723 (38.2606, 20.28) -> (38.2606, 20.816) construction
  spline S868 degree 3 poles (38.2606, 23.3701) (38.2606, 23.9061) (37.826, 24.3407) (37.29, 24.3407) knots 0 0 0 0 1 1 1 1
  line L2724 (38.2606, 23.3701) -> (38.2606, 23.9061) construction
  line L2725 (38.2606, 23.9061) -> (37.826, 24.3407) construction
  line L2726 (37.826, 24.3407) -> (37.29, 24.3407) construction
  spline S869 degree 3 poles (37.29, 24.3407) (36.754, 24.3407) (36.3194, 23.9061) (36.3194, 23.3701) knots 0 0 0 0 1 1 1 1
  line L2727 (37.29, 24.3407) -> (36.754, 24.3407) construction
  line L2728 (36.754, 24.3407) -> (36.3194, 23.9061) construction
  line L2729 (36.3194, 23.9061) -> (36.3194, 23.3701) construction
  spline S870 degree 3 poles (36.3194, 23.3701) (36.3194, 22.8341) (36.754, 22.3996) (37.29, 22.3996) knots 0 0 0 0 1 1 1 1
  line L2730 (36.3194, 23.3701) -> (36.3194, 22.8341) construction
  line L2731 (36.3194, 22.8341) -> (36.754, 22.3996) construction
  line L2732 (36.754, 22.3996) -> (37.29, 22.3996) construction
  spline S871 degree 3 poles (37.29, 22.3996) (37.826, 22.3996) (38.2606, 22.8341) (38.2606, 23.3701) knots 0 0 0 0 1 1 1 1
  line L2733 (37.29, 22.3996) -> (37.826, 22.3996) construction
  line L2734 (37.826, 22.3996) -> (38.2606, 22.8341) construction
  line L2735 (38.2606, 22.8341) -> (38.2606, 23.3701) construction
  spline S872 degree 3 poles (38.2606, 25.9242) (38.2606, 26.4602) (37.826, 26.8948) (37.29, 26.8948) knots 0 0 0 0 1 1 1 1
  line L2736 (38.2606, 25.9242) -> (38.2606, 26.4602) construction
  line L2737 (38.2606, 26.4602) -> (37.826, 26.8948) construction
  line L2738 (37.826, 26.8948) -> (37.29, 26.8948) construction
  spline S873 degree 3 poles (37.29, 26.8948) (36.754, 26.8948) (36.3194, 26.4602) (36.3194, 25.9242) knots 0 0 0 0 1 1 1 1
  line L2739 (37.29, 26.8948) -> (36.754, 26.8948) construction
  line L2740 (36.754, 26.8948) -> (36.3194, 26.4602) construction
  line L2741 (36.3194, 26.4602) -> (36.3194, 25.9242) construction
  spline S874 degree 3 poles (36.3194, 25.9242) (36.3194, 25.3882) (36.754, 24.9537) (37.29, 24.9537) knots 0 0 0 0 1 1 1 1
  line L2742 (36.3194, 25.9242) -> (36.3194, 25.3882) construction
  line L2743 (36.3194, 25.3882) -> (36.754, 24.9537) construction
  line L2744 (36.754, 24.9537) -> (37.29, 24.9537) construction
  spline S875 degree 3 poles (37.29, 24.9537) (37.826, 24.9537) (38.2606, 25.3882) (38.2606, 25.9242) knots 0 0 0 0 1 1 1 1
  line L2745 (37.29, 24.9537) -> (37.826, 24.9537) construction
  line L2746 (37.826, 24.9537) -> (38.2606, 25.3882) construction
  line L2747 (38.2606, 25.3882) -> (38.2606, 25.9242) construction
  spline S876 degree 3 poles (38.2606, 28.4784) (38.2606, 29.0143) (37.826, 29.4489) (37.29, 29.4489) knots 0 0 0 0 1 1 1 1
  line L2748 (38.2606, 28.4784) -> (38.2606, 29.0143) construction
  line L2749 (38.2606, 29.0143) -> (37.826, 29.4489) construction
  line L2750 (37.826, 29.4489) -> (37.29, 29.4489) construction
  spline S877 degree 3 poles (37.29, 29.4489) (36.754, 29.4489) (36.3194, 29.0143) (36.3194, 28.4784) knots 0 0 0 0 1 1 1 1
  line L2751 (37.29, 29.4489) -> (36.754, 29.4489) construction
  line L2752 (36.754, 29.4489) -> (36.3194, 29.0143) construction
  line L2753 (36.3194, 29.0143) -> (36.3194, 28.4784) construction
  spline S878 degree 3 poles (36.3194, 28.4784) (36.3194, 27.9423) (36.754, 27.5078) (37.29, 27.5078) knots 0 0 0 0 1 1 1 1
  line L2754 (36.3194, 28.4784) -> (36.3194, 27.9423) construction
  line L2755 (36.3194, 27.9423) -> (36.754, 27.5078) construction
  line L2756 (36.754, 27.5078) -> (37.29, 27.5078) construction
  spline S879 degree 3 poles (37.29, 27.5078) (37.826, 27.5078) (38.2606, 27.9423) (38.2606, 28.4784) knots 0 0 0 0 1 1 1 1
  line L2757 (37.29, 27.5078) -> (37.826, 27.5078) construction
  line L2758 (37.826, 27.5078) -> (38.2606, 27.9423) construction
  line L2759 (38.2606, 27.9423) -> (38.2606, 28.4784) construction
  spline S880 degree 3 poles (38.2606, 31.0325) (38.2606, 31.5684) (37.826, 32.003) (37.29, 32.003) knots 0 0 0 0 1 1 1 1
  line L2760 (38.2606, 31.0325) -> (38.2606, 31.5684) construction
  line L2761 (38.2606, 31.5684) -> (37.826, 32.003) construction
  line L2762 (37.826, 32.003) -> (37.29, 32.003) construction
  spline S881 degree 3 poles (37.29, 32.003) (36.754, 32.003) (36.3194, 31.5684) (36.3194, 31.0325) knots 0 0 0 0 1 1 1 1
  line L2763 (37.29, 32.003) -> (36.754, 32.003) construction
  line L2764 (36.754, 32.003) -> (36.3194, 31.5684) construction
  line L2765 (36.3194, 31.5684) -> (36.3194, 31.0325) construction
  spline S882 degree 3 poles (36.3194, 31.0325) (36.3194, 30.4965) (36.754, 30.0619) (37.29, 30.0619) knots 0 0 0 0 1 1 1 1
  line L2766 (36.3194, 31.0325) -> (36.3194, 30.4965) construction
  line L2767 (36.3194, 30.4965) -> (36.754, 30.0619) construction
  line L2768 (36.754, 30.0619) -> (37.29, 30.0619) construction
  spline S883 degree 3 poles (37.29, 30.0619) (37.826, 30.0619) (38.2606, 30.4965) (38.2606, 31.0325) knots 0 0 0 0 1 1 1 1
  line L2769 (37.29, 30.0619) -> (37.826, 30.0619) construction
  line L2770 (37.826, 30.0619) -> (38.2606, 30.4965) construction
  line L2771 (38.2606, 30.4965) -> (38.2606, 31.0325) construction
  spline S884 degree 3 poles (45.9229, 0.3832) (45.9229, 0.9191) (45.4883, 1.3537) (44.9523, 1.3537) knots 0 0 0 0 1 1 1 1
  line L2772 (45.9229, 0.3832) -> (45.9229, 0.9191) construction
  line L2773 (45.9229, 0.9191) -> (45.4883, 1.3537) construction
  line L2774 (45.4883, 1.3537) -> (44.9523, 1.3537) construction
  spline S885 degree 3 poles (44.9523, 1.3537) (44.4163, 1.3537) (43.9818, 0.9191) (43.9818, 0.3832) knots 0 0 0 0 1 1 1 1
  line L2775 (44.9523, 1.3537) -> (44.4163, 1.3537) construction
  line L2776 (44.4163, 1.3537) -> (43.9818, 0.9191) construction
  line L2777 (43.9818, 0.9191) -> (43.9818, 0.3832) construction
  spline S886 degree 3 poles (43.9818, 0.3832) (43.9818, -0.1529) (44.4163, -0.5874) (44.9523, -0.5874) knots 0 0 0 0 1 1 1 1
  line L2778 (43.9818, 0.3832) -> (43.9818, -0.1529) construction
  line L2779 (43.9818, -0.1529) -> (44.4163, -0.5874) construction
  line L2780 (44.4163, -0.5874) -> (44.9523, -0.5874) construction
  spline S887 degree 3 poles (44.9523, -0.5874) (45.4883, -0.5874) (45.9229, -0.1529) (45.9229, 0.3832) knots 0 0 0 0 1 1 1 1
  line L2781 (44.9523, -0.5874) -> (45.4883, -0.5874) construction
  line L2782 (45.4883, -0.5874) -> (45.9229, -0.1529) construction
  line L2783 (45.9229, -0.1529) -> (45.9229, 0.3832) construction
  spline S888 degree 3 poles (48.477, 0.3832) (48.477, 0.9191) (48.0424, 1.3537) (47.5064, 1.3537) knots 0 0 0 0 1 1 1 1
  line L2784 (48.477, 0.3832) -> (48.477, 0.9191) construction
  line L2785 (48.477, 0.9191) -> (48.0424, 1.3537) construction
  line L2786 (48.0424, 1.3537) -> (47.5064, 1.3537) construction
  spline S889 degree 3 poles (47.5064, 1.3537) (46.9704, 1.3537) (46.5359, 0.9191) (46.5359, 0.3832) knots 0 0 0 0 1 1 1 1
  line L2787 (47.5064, 1.3537) -> (46.9704, 1.3537) construction
  line L2788 (46.9704, 1.3537) -> (46.5359, 0.9191) construction
  line L2789 (46.5359, 0.9191) -> (46.5359, 0.3832) construction
  spline S890 degree 3 poles (46.5359, 0.3832) (46.5359, -0.1529) (46.9704, -0.5874) (47.5064, -0.5874) knots 0 0 0 0 1 1 1 1
  line L2790 (46.5359, 0.3832) -> (46.5359, -0.1529) construction
  line L2791 (46.5359, -0.1529) -> (46.9704, -0.5874) construction
  line L2792 (46.9704, -0.5874) -> (47.5064, -0.5874) construction
  spline S891 degree 3 poles (47.5064, -0.5874) (48.0424, -0.5874) (48.477, -0.1529) (48.477, 0.3832) knots 0 0 0 0 1 1 1 1
  line L2793 (47.5064, -0.5874) -> (48.0424, -0.5874) construction
  line L2794 (48.0424, -0.5874) -> (48.477, -0.1529) construction
  line L2795 (48.477, -0.1529) -> (48.477, 0.3832) construction
  spline S892 degree 3 poles (47.3149, 9.7057) (47.3149, 10.9399) (46.3142, 11.9405) (45.08, 11.9405) knots 0 0 0 0 1 1 1 1
  line L2796 (47.3149, 9.7057) -> (47.3149, 10.9399) construction
  line L2797 (47.3149, 10.9399) -> (46.3142, 11.9405) construction
  line L2798 (46.3142, 11.9405) -> (45.08, 11.9405) construction
  spline S893 degree 3 poles (45.08, 11.9405) (43.8459, 11.9405) (42.8452, 10.9399) (42.8452, 9.7057) knots 0 0 0 0 1 1 1 1
  line L2799 (45.08, 11.9405) -> (43.8459, 11.9405) construction
  line L2800 (43.8459, 11.9405) -> (42.8452, 10.9399) construction
  line L2801 (42.8452, 10.9399) -> (42.8452, 9.7057) construction
  spline S894 degree 3 poles (42.8452, 9.7057) (42.8452, 8.4714) (43.8459, 7.4708) (45.08, 7.4708) knots 0 0 0 0 1 1 1 1
  line L2802 (42.8452, 9.7057) -> (42.8452, 8.4714) construction
  line L2803 (42.8452, 8.4714) -> (43.8459, 7.4708) construction
  line L2804 (43.8459, 7.4708) -> (45.08, 7.4708) construction
  spline S895 degree 3 poles (45.08, 7.4708) (46.3142, 7.4708) (47.3149, 8.4714) (47.3149, 9.7057) knots 0 0 0 0 1 1 1 1
  line L2805 (45.08, 7.4708) -> (46.3142, 7.4708) construction
  line L2806 (46.3142, 7.4708) -> (47.3149, 8.4714) construction
  line L2807 (47.3149, 8.4714) -> (47.3149, 9.7057) construction
  spline S896 degree 3 poles (53.5724, 9.7057) (53.5724, 10.8694) (52.6292, 11.8128) (51.4653, 11.8128) knots 0 0 0 0 1 1 1 1
  line L2808 (53.5724, 9.7057) -> (53.5724, 10.8694) construction
  line L2809 (53.5724, 10.8694) -> (52.6292, 11.8128) construction
  line L2810 (52.6292, 11.8128) -> (51.4653, 11.8128) construction
  spline S897 degree 3 poles (51.4653, 11.8128) (50.3018, 11.8128) (49.3582, 10.8694) (49.3582, 9.7057) knots 0 0 0 0 1 1 1 1
  line L2811 (51.4653, 11.8128) -> (50.3018, 11.8128) construction
  line L2812 (50.3018, 11.8128) -> (49.3582, 10.8694) construction
  line L2813 (49.3582, 10.8694) -> (49.3582, 9.7057) construction
  spline S898 degree 3 poles (49.3582, 9.7057) (49.3582, 8.542) (50.3018, 7.5984) (51.4653, 7.5984) knots 0 0 0 0 1 1 1 1
  line L2814 (49.3582, 9.7057) -> (49.3582, 8.542) construction
  line L2815 (49.3582, 8.542) -> (50.3018, 7.5984) construction
  line L2816 (50.3018, 7.5984) -> (51.4653, 7.5984) construction
  spline S899 degree 3 poles (51.4653, 7.5984) (52.6292, 7.5984) (53.5724, 8.542) (53.5724, 9.7057) knots 0 0 0 0 1 1 1 1
  line L2817 (51.4653, 7.5984) -> (52.6292, 7.5984) construction
  line L2818 (52.6292, 7.5984) -> (53.5724, 8.542) construction
  line L2819 (53.5724, 8.542) -> (53.5724, 9.7057) construction
  spline S900 degree 3 poles (50.316, 14.303) (50.316, 15.4314) (49.4011, 16.3463) (48.2727, 16.3463) knots 0 0 0 0 1 1 1 1
  line L2820 (50.316, 14.303) -> (50.316, 15.4314) construction
  line L2821 (50.316, 15.4314) -> (49.4011, 16.3463) construction
  line L2822 (49.4011, 16.3463) -> (48.2727, 16.3463) construction
  spline S901 degree 3 poles (48.2727, 16.3463) (47.1442, 16.3463) (46.2294, 15.4314) (46.2294, 14.303) knots 0 0 0 0 1 1 1 1
  line L2823 (48.2727, 16.3463) -> (47.1442, 16.3463) construction
  line L2824 (47.1442, 16.3463) -> (46.2294, 15.4314) construction
  line L2825 (46.2294, 15.4314) -> (46.2294, 14.303) construction
  spline S902 degree 3 poles (46.2294, 14.303) (46.2294, 13.1746) (47.1442, 12.2598) (48.2727, 12.2598) knots 0 0 0 0 1 1 1 1
  line L2826 (46.2294, 14.303) -> (46.2294, 13.1746) construction
  line L2827 (46.2294, 13.1746) -> (47.1442, 12.2598) construction
  line L2828 (47.1442, 12.2598) -> (48.2727, 12.2598) construction
  spline S903 degree 3 poles (48.2727, 12.2598) (49.4011, 12.2598) (50.316, 13.1746) (50.316, 14.303) knots 0 0 0 0 1 1 1 1
  line L2829 (48.2727, 12.2598) -> (49.4011, 12.2598) construction
  line L2830 (49.4011, 12.2598) -> (50.316, 13.1746) construction
  line L2831 (50.316, 13.1746) -> (50.316, 14.303) construction
  spline S904 degree 3 poles (10.1653, 0.3832) (10.1653, 0.9191) (9.7308, 1.3537) (9.1948, 1.3537) knots 0 0 0 0 1 1 1 1
  line L2832 (10.1653, 0.3832) -> (10.1653, 0.9191) construction
  line L2833 (10.1653, 0.9191) -> (9.7308, 1.3537) construction
  line L2834 (9.7308, 1.3537) -> (9.1948, 1.3537) construction
  spline S905 degree 3 poles (9.1948, 1.3537) (8.6588, 1.3537) (8.2242, 0.9191) (8.2242, 0.3832) knots 0 0 0 0 1 1 1 1
  line L2835 (9.1948, 1.3537) -> (8.6588, 1.3537) construction
  line L2836 (8.6588, 1.3537) -> (8.2242, 0.9191) construction
  line L2837 (8.2242, 0.9191) -> (8.2242, 0.3832) construction
  spline S906 degree 3 poles (8.2242, 0.3832) (8.2242, -0.1529) (8.6588, -0.5874) (9.1948, -0.5874) knots 0 0 0 0 1 1 1 1
  line L2838 (8.2242, 0.3832) -> (8.2242, -0.1529) construction
  line L2839 (8.2242, -0.1529) -> (8.6588, -0.5874) construction
  line L2840 (8.6588, -0.5874) -> (9.1948, -0.5874) construction
  spline S907 degree 3 poles (9.1948, -0.5874) (9.7308, -0.5874) (10.1653, -0.1529) (10.1653, 0.3832) knots 0 0 0 0 1 1 1 1
  line L2841 (9.1948, -0.5874) -> (9.7308, -0.5874) construction
  line L2842 (9.7308, -0.5874) -> (10.1653, -0.1529) construction
  line L2843 (10.1653, -0.1529) -> (10.1653, 0.3832) construction
  spline S908 degree 3 poles (12.7194, 0.3832) (12.7194, 0.9191) (12.2849, 1.3537) (11.7489, 1.3537) knots 0 0 0 0 1 1 1 1
  line L2844 (12.7194, 0.3832) -> (12.7194, 0.9191) construction
  line L2845 (12.7194, 0.9191) -> (12.2849, 1.3537) construction
  line L2846 (12.2849, 1.3537) -> (11.7489, 1.3537) construction
  spline S909 degree 3 poles (11.7489, 1.3537) (11.2129, 1.3537) (10.7783, 0.9191) (10.7783, 0.3832) knots 0 0 0 0 1 1 1 1
  line L2847 (11.7489, 1.3537) -> (11.2129, 1.3537) construction
  line L2848 (11.2129, 1.3537) -> (10.7783, 0.9191) construction
  line L2849 (10.7783, 0.9191) -> (10.7783, 0.3832) construction
  spline S910 degree 3 poles (10.7783, 0.3832) (10.7783, -0.1529) (11.2129, -0.5874) (11.7489, -0.5874) knots 0 0 0 0 1 1 1 1
  line L2850 (10.7783, 0.3832) -> (10.7783, -0.1529) construction
  line L2851 (10.7783, -0.1529) -> (11.2129, -0.5874) construction
  line L2852 (11.2129, -0.5874) -> (11.7489, -0.5874) construction
  spline S911 degree 3 poles (11.7489, -0.5874) (12.2849, -0.5874) (12.7194, -0.1529) (12.7194, 0.3832) knots 0 0 0 0 1 1 1 1
  line L2853 (11.7489, -0.5874) -> (12.2849, -0.5874) construction
  line L2854 (12.2849, -0.5874) -> (12.7194, -0.1529) construction
  line L2855 (12.7194, -0.1529) -> (12.7194, 0.3832) construction
  spline S912 degree 3 poles (15.2735, 0.3832) (15.2735, 0.9191) (14.839, 1.3537) (14.303, 1.3537) knots 0 0 0 0 1 1 1 1
  line L2856 (15.2735, 0.3832) -> (15.2735, 0.9191) construction
  line L2857 (15.2735, 0.9191) -> (14.839, 1.3537) construction
  line L2858 (14.839, 1.3537) -> (14.303, 1.3537) construction
  spline S913 degree 3 poles (14.303, 1.3537) (13.767, 1.3537) (13.3324, 0.9191) (13.3324, 0.3832) knots 0 0 0 0 1 1 1 1
  line L2859 (14.303, 1.3537) -> (13.767, 1.3537) construction